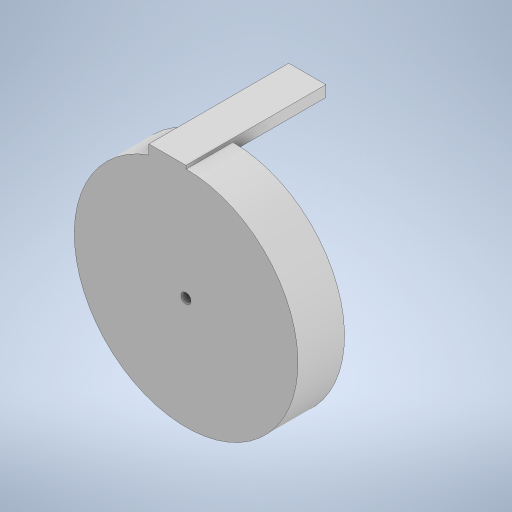
# Autodesk Inventor part: Disc
Saved by Autodesk Inventor 2023 (Build 270158000, 158)
## iProperties
Created: 2023-04-27
Part Number: Disc
Material: Generic
Document SubType Name: Modeling
Designer: alexa
Density: 1 g/cm^3
Appearance: Default
Author: alexa
Autodesk Inventor part; units mm, degrees
ref_plane "YZ Plane" through (0, 0, 0) normal (1, 0, 0) x (0, 1, 0)
ref_plane "XZ Plane" through (0, 0, 0) normal (0, 1, 0) x (-1, 0, 0)
ref_plane "XY Plane" through (0, 0, 0) normal (0, 0, 1) x (1, 0, 0)
sketch "Sketch1" plane through (0, 0, 0) normal (0, 0, 1) x (1, 0, 0)
  circle A0 centre (0, 0) radius 60
  circle A1 centre (0, 0) radius 2.65
  dimension "d0" = 120
  dimension "d1" = 5.3
  constraints: 2 centre point, 2 coincident
  measures "d0" diameter of A0
  measures "d1" diameter of A1
extrude "Extrusion1" add sketch "Sketch1" along normal blind 5
sketch "Sketch4" plane through (0, 0, 0) normal (0, 0, -1) x (-1, 0, 0)
  circle A0 centre (0, 0) radius 2.65 projected
  circle A1 centre (0, 0) radius 54.85
  circle A2 centre (0, 0) radius 60
  dimension "d13" = 109.7
  dimension "d14" = 120
  constraints: 2 centre point, 2 coincident
  measures "d13" diameter of A1
  measures "d14" diameter of A2
extrude "Extrusion4" add sketch "Sketch4" along normal blind 20 contours A2
sketch "Sketch7" plane through (0, 0, -20) normal (0, 0, -1) x (-1, 0, 0)
  circle A0 centre (0, 0) radius 54.85 projected
  line L0 (0, 54.85) -> (30.5637, 54.85)
  line L1 (30.5637, 54.85) -> (30.5637, 55.75)
  line L2 (30.5637, 55.75) -> (0, 55.75)
  line L3 (0, 55.75) -> (0, 54.85)
  line L4 (18, 55.75) -> (18, 54.85)
  line L5 (4.9967, 54.85) -> (4.9967, 54.185)
  line L6 (4.9967, 54.185) -> (0, 54.85)
  dimension "d25" = 0.9
  constraints: 14 end point, 5 perpendicular, 3 point on line, 2 horizontal, 1 vertical alignment, 1 other
  measures "d25" distance of L0.end L1.end
extrude "Extrusion7" cut sketch "Sketch7" against normal blind 20 contours L0 L5 A0 | L3 L2 L4 L0 | A0 L5 L6 picked at (2.2214, 54.6199)
sketch "Sketch8" plane through (0, 0, -20) normal (0, 0, -1) x (-1, 0, 0)
  arc A0 (0, 54.85) -> (4.9967, 54.6219) centre (0, 0) ccw projected
  line L0 (19.9252, 51.1029) -> (19.9252, 61.7106)
  line L1 (19.9252, 61.7106) -> (0, 61.7106)
  line L2 (0, 55.75) -> (18, 55.75) projected
  line L3 (0, 61.7106) -> (0, 55.75)
  line L4 (0, 55.75) -> (18, 55.75)
  line L5 (18, 55.75) -> (18, 54.85) projected
  line L6 (18, 55.75) -> (18, 54.85)
  line L7 (18, 54.85) -> (4.9967, 54.85)
  line L8 (4.9967, 54.85) -> (4.9967, 54.6219) projected
  line L9 (4.9967, 54.85) -> (4.9967, 54.6219)
  line L10 (18, 54.85) -> (4.9967, 54.85) projected
  line L11 (7.5379, 54.85) -> (7.5379, 54.3296)
  arc A1 (19.9685, 51.6391) -> (7.5379, 54.85) centre (0, 0) ccw
  line L12 (9.6264, 54.85) -> (9.6264, 54.5222)
  point P0 (19.9252, 51.6559)
  constraints: 18 end point, 6 perpendicular, 5 point on circle, 2 point on line, 2 vertical, 1 centre point, 1 coincident, 1 collinear
extrude "Extrusion8" add sketch "Sketch8" along normal blind 50 and the other way blind 25 contours A1 L12 L7 L5 L2 L3 L1 L0
chamfer "Chamfer1" distance 0.5 angle 45 1 edges at (-14.8452, 53.3382, -20)
sketch "Sketch9" plane through (0, 0, -20) normal (0, 0, -1) x (-1, 0, 0)
  line L0 (9.6264, 54.0144) -> (9.6264, 54.85) projected
  line L1 (9.6264, 54.85) -> (4.9967, 54.85) projected
  line L2 (9.6264, 54.85) -> (4.9967, 54.85)
  line L3 (4.9967, 54.85) -> (4.9967, 54.6219) projected
  line L4 (4.9967, 54.85) -> (4.9967, 54.6219)
  line L5 (4.9967, 54.6219) -> (4.9967, 54.2488)
  line L6 (4.9967, 54.2488) -> (9.6264, 53.9987)
  arc A0 (0, 54.85) -> (4.9967, 54.6219) centre (0, 0) ccw projected
  line L7 (9.6264, 54.85) -> (9.6264, 53.9987)
  constraints: 10 end point, 1 horizontal, 1 parallel, 1 perpendicular, 1 point on circle, 1 point on line
extrude "Extrusion9" cut sketch "Sketch9" against normal blind 20
body "Solid1"
